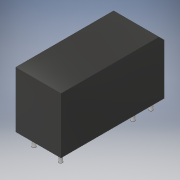
# Autodesk Inventor part: RZ03-1A4-D005
Saved by Autodesk Inventor 2018 (Build 220112000, 112)
## iProperties
Created: 2018-02-28
Part Number: RZ03-1A4-D005
Material: Generic
Document SubType Name: Modeling
Designer: brutu
Density: 1 g/cm^3
Appearance: Dark Gray
Author: brutu
Autodesk Inventor part; units mm, degrees
ref_plane "YZ Plane" through (0, 0, 0) normal (1, 0, 0) x (0, 1, 0)
ref_plane "XZ Plane" through (0, 0, 0) normal (0, 1, 0) x (-1, 0, 0)
ref_plane "XY Plane" through (0, 0, 0) normal (0, 0, 1) x (1, 0, 0)
sketch "Sketch1" plane through (0, 0, 0) normal (0, 1, 0) x (-1, 0, 0)
  line L0 (6.35, 14.5) -> (-6.35, 14.5)
  line L1 (-6.35, 14.5) -> (-6.35, -14.5)
  line L2 (-6.35, -14.5) -> (6.35, -14.5)
  line L3 (6.35, -14.5) -> (6.35, 14.5)
  point P0 (0, 0)
  dimension "d0" = 29
  dimension "d1" = 12.7
  dimension "d2" = 6.35
  dimension "d3" = 14.5
  constraints: 8 end point, 2 parallel, 1 horizontal, 1 perpendicular
  measures "d0" distance of L2.end L0.start
  measures "d1" distance of L0.start L0.end
  measures "d2" distance from line of point (0, 0) L3
  measures "d3" distance from line of point (0, 0) L0
extrude "Extrusion1" add sketch "Sketch1" along normal blind 15.7
sketch "Sketch2" plane through (0, 0, 0) normal (0, -1, 0) x (1, 0, 0)
  line L0 (-6.35, 14.5) -> (6.35, 14.5) projected
  line L1 (-6.35, -14.5) -> (-6.35, 14.5) projected
  line L2 (6.35, -14.5) -> (-6.35, -14.5) projected
  line L3 (6.35, 14.5) -> (6.35, -14.5) projected
  circle A0 centre (3.75, -13.36) radius 0.5
  circle A1 centre (-3.75, -8.32) radius 0.5
  circle A2 centre (3.75, -8.32) radius 0.5
  circle A3 centre (-3.75, -13.36) radius 0.5
  circle A4 centre (3.75, 11.98) radius 0.5
  circle A5 centre (-3.75, 11.98) radius 0.5
  point P0 (0, 0)
  dimension "d9" = 1
  dimension "d10" = 1
  dimension "d11" = 1
  dimension "d12" = 1
  dimension "d15" = 5.04
  dimension "d17" = 7.5
  dimension "d18" = 3.75
  dimension "d19" = 1
  dimension "d20" = 1
  dimension "d22" = 20.3
  dimension "d28" = 2.52
  constraints: 6 centre point, 4 vertical alignment, 3 horizontal alignment
  measures "d9" diameter of A2
  measures "d10" diameter of A0
  measures "d11" diameter of A1
  measures "d12" diameter of A3
  measures "d15" distance of A0.centre A2.centre
  measures "d17" distance of A1.centre A2.centre
  measures "d18" horizontal distance of A2.centre point (0, 0)
  measures "d19" diameter of A4
  measures "d20" diameter of A5
  measures "d22" distance of A4.centre A2.centre
  measures "d28" distance from line of L0 A4.centre
extrude "Extrusion2" add sketch "Sketch2" along normal blind 3.5 contours A0 | A1 | A2 | A3 | A4 | A5
chamfer "Chamfer2" distance 1.524 angle 45 1 edges at (0, 15.7, -14.5)
equation "\"d2\" = 0.5 * d1"
equation "\"d3\" = 0.5 * d0"
equation "\"d10\" = d9"
equation "\"d11\" = d9"
equation "\"d12\" = d9"
equation "\"d18\" = 0.5 * d17"
equation "\"d19\" = d9"
equation "\"d20\" = d9"
body "Solid1"
